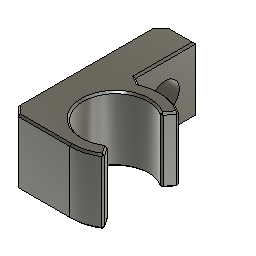
Staenderbohrmaschine Schluessel v1 (Autodesk Fusion 360 design; units mm, degrees)
Autodesk Fusion 360 part; units mm, degrees
sketch "Sketch1" plane through (0, 0, 0) normal (0, 0, 1) x (1, 0, 0)
  line L0 (0, 0) -> (8, 0)
  line L1 (8, 0) -> (8, 35)
  line L2 (8, 35) -> (0, 35)
  line L3 (0, 35) -> (0, 0)
  circle A0 centre (14, 10.5) radius 7.5
  circle A1 centre (14, 10.5) radius 10.5
  line L4 (8, 0) -> (14, 0)
  line L5 (18.3018, 16.6436) -> (20.0226, 19.1011)
  line L6 (18.3018, 4.3564) -> (20.0226, 1.8989)
  dimension "d1" = 15
  dimension "d2" = 3
  dimension "d3" = 8
  dimension "d4" = 14
  dimension "d5" = 35
  dimension "d6" = 110
  constraint horizontal L0
  constraint vertical L1
  constraint horizontal L2
  constraint vertical L3
  constraint coincident L0.start L3.end
  constraint concentric A0 A1
  constraint perpendicular L1 L4
  constraint tangent A1 L4
  constraint coincident A1 L4.end
  constraint coincident A0 L5.start
  constraint coincident A1 L5.end
  constraint coincident A0 L6.start
  constraint coincident A1 L6.end
  constraint coincident A0.centre L6
  constraint coincident A0.centre L5
  constraint vertical L5.start L6.start
  measures "d1" diameter of A0
  measures "d2" distance of A0 A1
  measures "d3" distance of L0.start L0.end
  measures "d4" horizontal distance of L0.start A0.centre
  measures "d5" distance of L0.start L2.end
  measures "d6" angle of L5 L6
sketch "Sketch3" plane through (0, 0, 0) normal (1, 0, 0) x (0, 1, 0)
  circle A0 centre (28, 0) radius 3.25
  dimension "d9" = 28
  dimension "d10" = 6.5
  constraint horizontal A0.centre origin
  measures "d9" distance of A0.centre origin
  measures "d10" diameter of A0
extrude "Extrude1" add sketch "Sketch1" along normal mid plane 15 contours L0 L1 L2 L3 A1 | L1 A1 L4 | L1 A0 A1 | L1 A0 A1 L6 | L1 A0 A1 L5
extrude "Extrude2" cut sketch "Sketch3" along normal up to surface (8 mm away)
chamfer "Chamfer1" distance 2 angle 45 3 edges at (0, 0, 0) (8, 19.1168, 0) (0, 35, 0)
chamfer "Chamfer2" distance 0.4 angle 45 4 edges at (20.0226, 1.8989, 0) (18.3018, 16.6436, 0) (18.3018, 4.3564, 0) (20.0226, 19.1011, 0) 2 faces at (2.2717, 15.8837, 7.5) (2.2717, 15.8837, -7.5)
